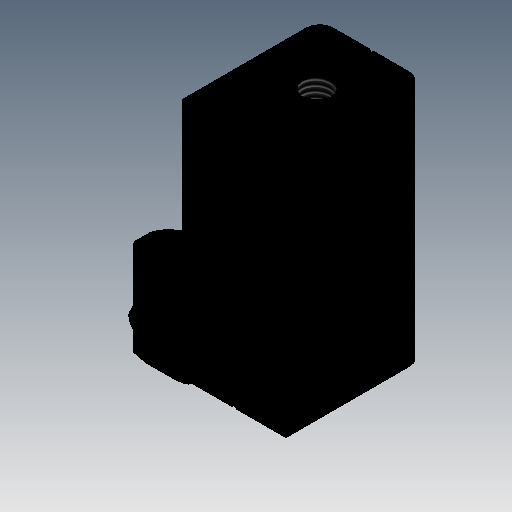
# Autodesk Inventor part: HCBRB8-45
Saved by Autodesk Inventor 2020 (Build 240168000, 168)
## iProperties
Part Number: HCBRB8-45
Material: 一般
Catalog Web Link: www.cadenas.de
Description: HCBR, HCBRB-Panel Support Brackets - Resin Type - for Center Mounting (One-Touch Mounting)
Vendor: MISUMI
Document SubType Name: Modeling
Designer: partserver
Manufacturer: MISUMI
Mass: 9.54612 g
Surface Area: 48.477 cm^2
Volume: 9.54612 cm^3
Density: 1 g/cm^3
Appearance: PSOLRGB-0-0-0
Category: PARTsolutions
Company: MISUMI
PSOL_IDENT_0: {$CADENAS_DATA\23d-libs\misumi\metric\39_accessories_for_al_extrusions\hcbr.prj},168 {VTYP=3D},{NB=H
PSOL_IDENT_1: CBRB8-45},{LINA=HCBRB8-45},{NN=HCBR, HCBRB},{DATE=08.06.2021 06:07:33},{GEOMDATE=12.08.2016 06:28:00
PSOL_IDENT_2: },{VERSION=},{LINEID=50},{WBVAR=COLOR},{WBNUMERIC=}  {NB=HCBRB8-45},{LINA=HCBRB8-45},{KT=DUMMY},{PN=
PSOL_IDENT_3: HCBRB8-45},{COLOR=B},{TS=HCBR},{MAT=Polyamide},{NO=8-45},{MASS=13.2},{A=35},{DIFF=5},{COL=0.00,0.00,
PSOL_IDENT_4: 0.00,0.00},{M=5},{KDM=4.134}
NB: HCBRB8-45
NN: HCBR, HCBRB
NT: Panel Support Brackets - Resin Type - for Center Mounting (One-Touch Mounting)
NBSYN: $PN.
LINA: HCBRB8-45
CATALOG: Misumi
PN: HCBRB8-45
COLOR: Black
MAT: Polyamide
NO: 8-45
MASS: 13.2
A: 35
DIFF: 5
SUPPLIER: MISUMI
ARTICLENO: HCBRB8-45
BOMINFO: HCBRB8-45
CREATOR: CADENAS GmbH
Title: HCBRB8-45
Author: Cadenas PARTsolutions
Comments: Panel Support Brackets - Resin Type - for Center Mounting (One-Touch Mounting)
Autodesk Inventor part; units mm, degrees
ref_plane "YZ Plane" through (0, 0, 0) normal (1, 0, 0) x (0, 1, 0)
ref_plane "XZ Plane" through (0, 0, 0) normal (0, 1, 0) x (-1, 0, 0)
ref_plane "XY Plane" through (0, 0, 0) normal (0, 0, 1) x (1, 0, 0)
sketch "Sketch_1" plane through (0, 0, 0) normal (0, 0, 1) x (1, 0, 0)
  line L0 (0, 28.35) -> (0, 10.45)
  line L1 (0, 10.45) -> (15, 10.45)
  line L2 (15, 10.45) -> (15, 28.35)
  arc A0 (15, 28.35) -> (13, 30.35) centre (13, 28.35) ccw
  line L3 (13, 30.35) -> (2, 30.35)
  arc A1 (2, 30.35) -> (0, 28.35) centre (2, 28.35) ccw
  constraints: 8 end point, 4 point on circle, 2 centre point
extrude "Extrusion1" add sketch "Sketch_1" against normal blind 35
sketch "Sketch_6" plane through (7.5, 0, 0) normal (1, 0, 0) x (0, 0, -1)
  line L0 (0, 21.9) -> (35, 21.9)
  line L1 (35, 21.9) -> (35, 18.65)
  line L2 (35, 18.65) -> (34.5, 19.15)
  line L3 (34.5, 19.15) -> (0.5, 19.15)
  line L4 (0.5, 19.15) -> (0, 18.65)
  line L5 (0, 18.65) -> (0, 21.9)
  line L6 (0, 21.9) -> (35, 21.9)
  constraints: 14 end point
revolve "Revolution1" cut sketch "Sketch_6" angle 360 about axis through (7.5, 21.9, 0) along (0, 0, 1)
sketch "Sketch_4" plane through (7.5, 0, 0) normal (1, 0, 0) x (0, 0, -1)
  line L0 (0, 23) -> (35, 23)
  line L1 (35, 23) -> (35, 19.75)
  line L2 (35, 19.75) -> (34.5, 20.25)
  line L3 (34.5, 20.25) -> (0.5, 20.25)
  line L4 (0.5, 20.25) -> (0, 19.75)
  line L5 (0, 19.75) -> (0, 23)
  line L6 (0, 23) -> (35, 23)
  constraints: 14 end point
revolve "Revolution2" cut sketch "Sketch_4" angle 360 about axis through (7.5, 23, 0) along (0, 0, 1)
sketch "Sketch_8" plane through (0, 22.45, 0) normal (0, 1, 0) x (1, 0, 0)
  line L0 (4.25, 0) -> (10.75, 0)
  line L1 (10.75, 0) -> (10.25, 0.5)
  line L2 (10.25, 0.5) -> (10.25, 34.5)
  line L3 (10.25, 34.5) -> (10.75, 35)
  line L4 (10.75, 35) -> (4.25, 35)
  line L5 (4.25, 35) -> (4.75, 34.5)
  line L6 (4.75, 34.5) -> (4.75, 0.5)
  line L7 (4.75, 0.5) -> (4.25, 0)
  constraints: 16 end point
extrude "Extrusion2" cut sketch "Sketch_8" along normal mid plane 1.1
sketch "Sketch_10" plane through (0, 0, -0.5) normal (0, 0, 1) x (1, 0, 0)
  arc A0 (4.75, 21.9) -> (10.25, 21.9) centre (7.5, 21.9) ccw
  line L0 (10.25, 21.9) -> (10.25, 23)
  arc A1 (10.25, 23) -> (4.75, 23) centre (7.5, 23) ccw
  line L1 (4.75, 23) -> (4.75, 21.9)
  constraints: 4 end point, 4 point on circle, 2 centre point
extrude "Extrusion3" add sketch "Sketch_10" against normal blind 34
sketch "Sketch_11" plane through (7.5, 0, 0) normal (1, 0, 0) x (0, 0, -1)
  line L0 (0.5, 22.45) -> (34.5, 22.45)
  line L1 (34.5, 22.45) -> (34.5, 19.95)
  line L2 (34.5, 19.95) -> (34.067, 20.383)
  line L3 (34.067, 20.383) -> (0.933, 20.383)
  line L4 (0.933, 20.383) -> (0.5, 19.95)
  line L5 (0.5, 19.95) -> (0.5, 22.45)
  line L6 (0.5, 22.45) -> (34.5, 22.45)
  constraints: 14 end point
revolve "Revolution3" cut sketch "Sketch_11" angle 360 about axis through (7.5, 22.45, -0.5) along (0, 0, 1)
thread "Thread1" size "M5x0.8" class "6H" standard "ISO Metric profile" full length
sketch "Sketch_2" plane through (7.5, 0, 0) normal (1, 0, 0) x (0, 0, -1)
  line L0 (7.9, 4.25) -> (7.9, 1.8)
  line L1 (7.9, 1.8) -> (10.15, 0)
  line L2 (10.15, 0) -> (23.65, 0)
  line L3 (23.65, 0) -> (25.9, 1.8)
  line L4 (25.9, 1.8) -> (25.9, 4.25)
  line L5 (25.9, 4.25) -> (22.9, 4.25)
  line L6 (22.9, 4.25) -> (22.9, 10.45)
  line L7 (22.9, 10.45) -> (12.1, 10.45)
  line L8 (12.1, 10.45) -> (12.1, 4.25)
  line L9 (12.1, 4.25) -> (7.9, 4.25)
  constraints: 20 end point
extrude "Extrusion4" add sketch "Sketch_2" along normal mid plane 8.45
sketch "Sketch_3" plane through (7.5, 0, 0) normal (1, 0, 0) x (0, 0, -1)
  line L0 (17.5, 0) -> (17.5, -3.15)
  line L1 (17.5, -3.15) -> (15.8, -3.15)
  line L2 (15.8, -3.15) -> (14.25, 0)
  line L3 (14.25, 0) -> (17.5, 0)
  line L4 (17.5, 0) -> (17.5, -3.15)
  constraints: 10 end point
revolve "Revolution4" add sketch "Sketch_3" angle 360 about axis through (7.5, 0, -17.5) along (0, 1, 0)
sketch "Sketch_12" plane through (0, 0, 0) normal (0, 1, 0) x (-1, 0, 0)
  line L0 (-2.275, -6.5) -> (-11.725, -6.5)
  line L1 (-11.725, -6.5) -> (-11.725, -7.5)
  line L2 (-11.725, -7.5) -> (-10.225, -7.5)
  arc A0 (-3.275, -10.5) -> (-10.225, -7.5) centre (-10.4183, -17.4981) ccw
  line L3 (-3.275, -10.5) -> (-2.275, -10.5)
  line L4 (-2.275, -10.5) -> (-2.275, -6.5)
  constraints: 10 end point, 2 point on circle, 1 centre point
extrude "Extrusion5" cut sketch "Sketch_12" along normal mid plane 16
sketch "Sketch_13" plane through (0, 0, 0) normal (0, 1, 0) x (-1, 0, 0)
  line L0 (-3.275, -26.9) -> (-3.275, -25.9)
  line L1 (-3.275, -25.9) -> (-4.775, -25.9)
  arc A0 (-11.725, -23.9) -> (-4.775, -25.9) centre (-5.6717, -15.9403) ccw
  line L2 (-11.725, -23.9) -> (-12.725, -23.9)
  line L3 (-12.725, -23.9) -> (-12.725, -26.9)
  line L4 (-12.725, -26.9) -> (-3.275, -26.9)
  constraints: 10 end point, 2 point on circle, 1 centre point
extrude "Extrusion6" cut sketch "Sketch_13" along normal mid plane 16
sketch "Sketch_7" plane through (15, 0, 0) normal (1, 0, 0) x (0, 0, -1)
  line L0 (2, 15.9) -> (2, 12.65)
  line L1 (2, 12.65) -> (16.5, 12.65)
  line L2 (16.5, 12.65) -> (16.5, 15.9)
  line L3 (16.5, 15.9) -> (2, 15.9)
  constraints: 8 end point
extrude "Extrusion7" cut sketch "Sketch_7" against normal blind 15
sketch "Sketch_5" plane through (15, 0, 0) normal (1, 0, 0) x (0, 0, -1)
  line L0 (18.5, 15.9) -> (18.5, 12.65)
  line L1 (18.5, 12.65) -> (33, 12.65)
  line L2 (33, 12.65) -> (33, 15.9)
  line L3 (33, 15.9) -> (18.5, 15.9)
  constraints: 8 end point
extrude "Extrusion8" cut sketch "Sketch_5" against normal blind 15
sketch "Sketch13" plane through (11.725, 0, 0) normal (1, 0, 0) x (0, 0, -1)
  point P0 (17.5, 5)
hole "Hole1" at (11.725, 5, -17.5) direction (-1, 0, 0) diameter 2 depth 0.3
sketch "Sketch_9" plane through (0, 0, 0) normal (0, 1, 0) x (-1, 0, 0)
  line L0 (0, -17.8) -> (0, -17.2)
  line L1 (0, -17.2) -> (-0.3, -17.5)
  line L2 (-0.3, -17.5) -> (0, -17.8)
  constraints: 6 end point
extrude "Extrusion9" cut sketch "Sketch_9" along normal blind 40
sketch "Sketch_15" plane through (0, 0, 0) normal (0, 1, 0) x (-1, 0, 0)
  line L0 (-14.7, -17.5) -> (-15, -17.2)
  line L1 (-15, -17.2) -> (-15, -17.8)
  line L2 (-15, -17.8) -> (-14.7, -17.5)
  constraints: 6 end point
extrude "Extrusion10" cut sketch "Sketch_15" along normal blind 40
sketch "Sketch_16" plane through (0, 0, 0) normal (0, 1, 0) x (-1, 0, 0)
  line L0 (-7.2, 0) -> (-7.8, 0)
  line L1 (-7.8, 0) -> (-7.5, -0.3)
  line L2 (-7.5, -0.3) -> (-7.2, 0)
  constraints: 6 end point
extrude "Extrusion11" cut sketch "Sketch_16" along normal blind 40
sketch "Sketch_17" plane through (0, 0, 0) normal (0, 1, 0) x (-1, 0, 0)
  line L0 (-7.2, -35) -> (-7.5, -34.7)
  line L1 (-7.5, -34.7) -> (-7.8, -35)
  line L2 (-7.8, -35) -> (-7.2, -35)
  constraints: 6 end point
extrude "Extrusion12" cut sketch "Sketch_17" along normal blind 40
sketch "Sketch_18" plane through (0, 4.25, 0) normal (0, 1, 0) x (1, 0, 0)
  line L0 (-2, 5) -> (18, 5)
  line L1 (18, 5) -> (18, 30)
  line L2 (18, 30) -> (-2, 30)
  line L3 (-2, 30) -> (-2, 5)
  line L4 (2.775, 22.9882) -> (2.775, 13.6781)
  line L5 (2.775, 13.6781) -> (12.225, 12.0118)
  line L6 (12.225, 12.0118) -> (12.225, 21.3219)
  line L7 (12.225, 21.3219) -> (2.775, 22.9882)
  constraints: 16 end point
extrude "Extrusion13" cut sketch "Sketch_18" along normal blind 6.2
sketch "Sketch_19" plane through (0, 4.25, 0) normal (0, 1, 0) x (1, 0, 0)
  line L0 (13.225, 30) -> (13.225, 5)
  line L1 (1.275, 5) -> (12.725, 5)
  line L2 (12.725, 5) -> (12.725, 11.9237)
  line L3 (12.725, 11.9237) -> (1.275, 13.9426)
  line L4 (1.275, 13.9426) -> (1.275, 5)
  constraints: 10 end point
revolve "Revolution5" cut sketch "Sketch_19" angle 10 about axis through (13.225, 4.25, -30) along (0, 0, 1)
sketch "Sketch_20" plane through (0, 4.25, 0) normal (0, 1, 0) x (1, 0, 0)
  line L0 (1.775, 5) -> (1.775, 30)
  line L1 (2.275, 30) -> (2.275, 23.0763)
  line L2 (2.275, 23.0763) -> (13.725, 21.0574)
  line L3 (13.725, 21.0574) -> (13.725, 30)
  line L4 (13.725, 30) -> (2.275, 30)
  constraints: 10 end point
revolve "Revolution6" cut sketch "Sketch_20" angle 10 about axis through (1.775, 4.25, -5) along (0, 0, -1)
body "Solid1"
